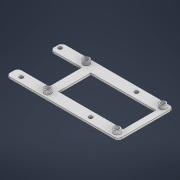
# Autodesk Inventor part: Adapter_Arduino
Saved by Autodesk Inventor 2021 (Build 250183000, 183)
## iProperties
Created: 2021-02-21
Part Number: Adapter_Arduino
Material: Generisch
Document SubType Name: Modeling
Designer: Ctroi
Density: 1 g/cm^3
Appearance: Vorgabe
Author: Ctroi
## iProperties of the stored document _3D-Druck.ipt
Created: 2021-02-21
Part Number: _3D-Druck
Material: Generisch
Document SubType Name: Modeling
Designer: Ctroi
Density: 1 g/cm^3
Appearance: Vorgabe
Author: Ctroi
Autodesk Inventor part; units mm, degrees
ref_plane "YZ Plane" through (0, 0, 0) normal (1, 0, 0) x (0, 1, 0)
ref_plane "XZ Plane" through (0, 0, 0) normal (0, 1, 0) x (-1, 0, 0)
ref_plane "XY Plane" through (0, 0, 0) normal (0, 0, 1) x (1, 0, 0)
sketch "Skizze1" plane through (0, 0, 0) normal (0, 1, 0) x (-1, 0, 0)
  line L0 (-65, 30) -> (65, 30)
  line L1 (65, 30) -> (65, -30)
  line L2 (65, -30) -> (-65, -30)
  line L3 (-65, -30) -> (-65, 30)
  line L4 (0, -42) -> (0, 42) projected
  line L5 (-91, 0) -> (91, 0) projected
  point P0 (0, 0)
  dimension "d0" = 130
  dimension "d1" = 60
  constraints: 8 end point, 2 parallel, 1 horizontal, 1 perpendicular, 2 other
  measures "d0" distance of L1.end L2.end
  measures "d1" distance of L0.end L1.end
extrude "Extrusion1" add sketch "Skizze1" along normal blind 2
sketch "Skizze2" plane through (0, 2, 0) normal (0, 1, 0) x (1, 0, 0)
  line L0 (0, 42) -> (0, -42) projected
  line L1 (91, 0) -> (-91, 0) projected
  circle A0 centre (49.76, -24.13) radius 2.25
  line L2 (65, -30) -> (65, 30) projected
  circle A1 centre (51.03, 24.13) radius 2.25
  circle A2 centre (-31.52, 24.13) radius 2.25
  circle A3 centre (-25.17, -24.13) radius 2.25
  circle A4 centre (21.3223, -24.13) radius 2
  circle A5 centre (22.5923, 24.13) radius 2
  circle A6 centre (-59.9577, 24.13) radius 2
  circle A7 centre (-53.6077, -24.13) radius 2
  line L3 (-65, 30) -> (-65, -30) projected
  circle A8 centre (49.76, -24.13) radius 3.5
  circle A9 centre (-25.17, -24.13) radius 3.5
  circle A10 centre (51.03, 24.13) radius 3.5
  circle A11 centre (-31.52, 24.13) radius 3.5
  point P0 (0, 0)
  dimension "d4" = 4.5
  dimension "d5" = 24.13
  dimension "d6" = 15.24
  dimension "d7" = 4.5
  dimension "d8" = 24.13
  dimension "d9" = 13.97
  dimension "d10" = 4.5
  dimension "d11" = 24.13
  dimension "d12" = 82.55
  dimension "d13" = 4.5
  dimension "d14" = 24.13
  dimension "d15" = 74.93
  dimension "d16" = 4
  dimension "d17" = 4
  dimension "d18" = 4
  dimension "d19" = 82.55
  dimension "d20" = 4
  dimension "d21" = 74.93
  dimension "d22" = 24.13
  dimension "d23" = 24.13
  dimension "d24" = 11.3923
  dimension "d25" = 5.0423
  dimension "d26" = 24.13
  dimension "d27" = 24.13
  dimension "d41" = 7
  dimension "d42" = 7
  dimension "d43" = 7
  dimension "d44" = 7
  constraints: 12 centre point, 4 coincident
  measures "d4" diameter of A0
  measures "d5" distance from line of L1 A0.centre
  measures "d6" distance from line of L2 A0.centre
  measures "d7" diameter of A1
  measures "d8" distance from line of L1 A1.centre
  measures "d9" distance from line of L2 A1.centre
  measures "d10" diameter of A2
  measures "d11" distance from line of L1 A2.centre
  measures "d12" distance of A1.centre A2.centre
  measures "d13" diameter of A3
  measures "d14" distance from line of L1 A3.centre
  measures "d15" distance of A0.centre A3.centre
  measures "d16" diameter of A4
  measures "d17" diameter of A5
  measures "d18" diameter of A6
  measures "d19" distance of A5.centre A6.centre
  measures "d20" diameter of A7
  measures "d21" distance of A4.centre A7.centre
  measures "d22" distance from line of L1 A4.centre
  measures "d23" distance from line of L1 A7.centre
  measures "d24" distance from line of L3 A7.centre
  measures "d25" distance from line of L3 A6.centre
  measures "d26" distance from line of L1 A6.centre
  measures "d27" distance from line of L1 A5.centre
  measures "d41" diameter of A8
  measures "d42" diameter of A9
  measures "d43" diameter of A10
  measures "d44" diameter of A11
extrude "Extrusion2" cut sketch "Skizze2" against normal up to surface (2 mm away) contours A0 | A1 | A2 | A3 | A4 | A5 | A6 | A7
sketch "Skizze3" plane through (0, 2, 0) normal (0, 1, 0) x (1, 0, 0)
  line L0 (-65, 30) -> (-65, -30) projected
  line L1 (-65, -17.5) -> (-30, -17.5)
  line L2 (-30, -17.5) -> (-30, 17.5)
  line L3 (-30, 17.5) -> (-65, 17.5)
  line L4 (-65, 17.5) -> (-65, -17.5)
  line L5 (91, 0) -> (-91, 0) projected
  line L6 (50, -17.5) -> (-20, -17.5)
  line L7 (-20, -17.5) -> (-20, 17.5)
  line L8 (-20, 17.5) -> (50, 17.5)
  line L9 (50, 17.5) -> (50, -17.5)
  line L10 (65, -30) -> (65, 30) projected
  point P0 (0, 0)
  dimension "d30" = 35
  dimension "d31" = 35
  dimension "d36" = 70
  dimension "d37" = 35
  dimension "d38" = 15
  constraints: 16 end point, 4 parallel, 2 horizontal, 2 perpendicular, 1 point on line, 2 other
  measures "d30" distance between parallel lines of L3 L1
  measures "d31" distance between parallel lines of L0 L2
  measures "d36" distance of L7.end L8.end
  measures "d37" distance of L6.end L7.end
  measures "d38" distance between parallel lines of L10 L9
extrude "Extrusion3" cut sketch "Skizze3" against normal up to surface (2 mm away)
sketch "Skizze4" plane through (-65, 0, 30) normal (-1, 0, 0) x (0, 0, 1)
  line L0 (-12.5, 2) -> (-12.5, 0) projected
  line L1 (0, 0) -> (-12.5, 0)
  line L2 (-12.5, 0) -> (-12.5, 2)
  line L3 (-12.5, 2) -> (0, 2)
  line L4 (0, 2) -> (0, 0)
  line L5 (-60, 0) -> (-60, 2) projected
  line L6 (-47.5, 0) -> (-47.5, 2) projected
  line L7 (-60, 0) -> (-47.5, 0)
  line L8 (-47.5, 0) -> (-47.5, 2)
  line L9 (-47.5, 2) -> (-60, 2)
  line L10 (-60, 2) -> (-60, 0)
  point P0 (-30, 0)
  constraints: 16 end point, 4 parallel, 2 horizontal, 2 perpendicular
extrude "Extrusion4" cut sketch "Skizze4" against normal blind 1
sketch "Skizze5" plane through (65, 0, 30) normal (1, 0, 0) x (0, 0, -1)
  line L0 (0, 0) -> (0, 2) projected
  line L1 (60, 0) -> (60, 2) projected
  line L2 (0, 2) -> (60, 2)
  line L3 (60, 2) -> (60, 0)
  line L4 (60, 0) -> (0, 0)
  line L5 (0, 0) -> (0, 2)
  point P0 (30, 0)
  constraints: 8 end point, 2 parallel, 1 horizontal, 1 perpendicular
extrude "Extrusion5" cut sketch "Skizze5" against normal blind 8
extrude "Extrusion6" add sketch "Skizze2" along normal blind 4 contours A8 | A9 | A10 | A11
fillet "Rundung1" radius 4 4 edges at (-64, 1, -30) (-64, 1, -17.5) (-64, 1, 17.5) (-64, 1, 30)
fillet "Rundung2" radius 4 2 edges at (57, 1, 30) (57, 1, -30)
